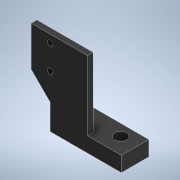
# Autodesk Inventor part: Endschalterhalter1
Saved by Autodesk Inventor 2021 (Build 250183000, 183)
## iProperties
Created: 2024-08-29
Part Number: Endschalterhalter1
Material: Generic
Document SubType Name: Modeling
Designer: Lukas
Density: 1 g/cm^3
Appearance: Default
Author: Lukas
Autodesk Inventor part; units mm, degrees
ref_plane "YZ Plane" through (0, 0, 0) normal (1, 0, 0) x (0, 1, 0)
ref_plane "XZ Plane" through (0, 0, 0) normal (0, 1, 0) x (-1, 0, 0)
ref_plane "XY Plane" through (0, 0, 0) normal (0, 0, 1) x (1, 0, 0)
sketch "Sketch1" plane through (0, 0, 0) normal (0, 0, 1) x (1, 0, 0)
  line L0 (-14.5, 22.5) -> (0.5, 22.5)
  line L1 (9.5, 0) -> (-9.5, 0)
  line L2 (-9.5, 0) -> (-9.5, 11.825)
  line L3 (-9.5, 11.825) -> (-14.5, 11.825)
  line L4 (-14.5, 11.825) -> (-14.5, 22.5)
  line L5 (9.5, 0) -> (9.5, 4)
  line L6 (9.5, 4) -> (0.5, 4)
  line L7 (0.5, 4) -> (0.5, 22.5)
  circle A0 centre (-9.5, 20.325) radius 0.75
  circle A1 centre (-9.5, 13.825) radius 0.75
  point P0 (0, 0)
  point P1 (0, 0)
  dimension "d1" = 4
  dimension "d2" = 22.5
  dimension "d3" = 1.5
  dimension "d4" = 13.825
  dimension "d5" = 6.5
  dimension "d6" = 2
  dimension "d7" = 5
  dimension "d8" = 24
  dimension "d9" = 15
  dimension "d10" = 5
  constraints: 16 end point, 5 perpendicular, 2 centre point, 2 coincident, 2 horizontal, 1 equal radius, 1 midpoint, 1 vertical, 1 vertical alignment
  measures "d1" distance of L1.start L5.end
  measures "d2" distance between parallel lines of L0 L1
  measures "d3" diameter of A0
  measures "d4" distance from line of L1 A1.centre
  measures "d5" distance of A0.centre A1.centre
  measures "d6" distance from line of A1.centre L3
  measures "d7" distance from line of L4 A1.centre
  measures "d8" distance between parallel lines of L4 L5
  measures "d9" distance of L0.start L0.end
  measures "d10" distance of L2.end L3.end
extrude "Extrusion1" add sketch "Sketch1" along normal blind 1.5
sketch "Sketch2" plane through (0, 0, 0) normal (0, 0, -1) x (-1, 0, 0)
  line L0 (-9.5, 4) -> (-0.5, 4) projected
  line L1 (9.5, 11.825) -> (9.5, 0) projected
  line L2 (-9.5, 4) -> (9.5, 4)
  line L3 (9.5, 4) -> (9.5, 0)
  line L4 (9.5, 0) -> (-9.5, 0)
  line L5 (-9.5, 0) -> (-9.5, 4)
  point P0 (0, 0)
  constraints: 8 end point, 2 parallel, 1 horizontal, 1 perpendicular
extrude "Extrusion2" add sketch "Sketch2" along normal blind 5.8
sketch "Sketch3" plane through (-9.5, 4, 0) normal (0, 1, 0) x (1, 0, 0)
  circle A0 centre (14.5, 2.8) radius 1.6
  line L0 (0.75, -1.5) -> (-0.75, -1.5) projected
  line L1 (0, 5.8) -> (19, 5.8) projected
  point P0 (9.5, 0)
  point P1 (0, -1.5)
  dimension "d15" = 14.5
  dimension "d16" = 3
  dimension "d17" = 3.2
  constraints: 1 centre point
  measures "d15" horizontal distance of A0.centre point (0, -1.5)
  measures "d16" distance from line of L1 A0.centre
  measures "d17" diameter of A0
extrude "Extrusion3" cut sketch "Sketch3" against normal through all
chamfer "Chamfer1" distance 5 angle 45 1 edges at (-9.5, 11.825, 0.75)
body "Solid1"
